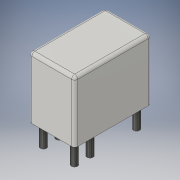
# Autodesk Inventor part: G5V-1-DC5_Relay
Saved by Autodesk Inventor 2016 (Build 200138000, 138)
## iProperties
Created: 2016-09-07
Part Number: G5V-1-DC5_Relay
Material: Generic
Document SubType Name: Modeling
Designer: jfixelle
Density: 1 g/cm^3
Appearance: White
Author: jfixelle
Autodesk Inventor part; units mm, degrees
ref_plane "YZ Plane" through (0, 0, 0) normal (1, 0, 0) x (0, 1, 0)
ref_plane "XZ Plane" through (0, 0, 0) normal (0, 1, 0) x (-1, 0, 0)
ref_plane "XY Plane" through (0, 0, 0) normal (0, 0, 1) x (1, 0, 0)
sketch "Sketch1" plane through (0, 0, 0) normal (0, 1, 0) x (-1, 0, 0)
  line L0 (3.75, 6.25) -> (-3.75, 6.25)
  line L1 (-3.75, 6.25) -> (-3.75, -6.25)
  line L2 (-3.75, -6.25) -> (3.75, -6.25)
  line L3 (3.75, -6.25) -> (3.75, 6.25)
  point P0 (0, 0)
  dimension "d0" = 7.5
  dimension "d1" = 3.75
  dimension "d2" = 12.5
  dimension "d3" = 6.25
  constraints: 8 end point, 2 parallel, 1 horizontal, 1 perpendicular
  measures "d0" distance of L1.end L2.end
  measures "d1" distance from line of point (0, 0) L3
  measures "d2" distance of L2.end L0.start
  measures "d3" distance from line of point (0, 0) L2
extrude "Extrusion1" add sketch "Sketch1" along normal blind 10
fillet "Fillet1" radius 0.5 8 edges at (3.75, 5, -6.25) (3.75, 5, 6.25) (-3.75, 5, 6.25) (0, 10, 6.25) (3.75, 10, 0) (0, 10, -6.25) (-3.75, 10, 0) (-3.75, 5, -6.25)
sketch "Sketch2" plane through (0, 0, 0) normal (0, -1, 0) x (1, 0, 0)
  circle A0 centre (2.54, 5.08) radius 0.5
  line L0 (3.75, 5.75) -> (3.75, -5.75) projected
  line L1 (3.75, 1.9877) -> (3.75, 0.9043)
  line L2 (1.2566, 6.25) -> (0.5094, 6.25)
  line L3 (-3.25, 6.25) -> (3.25, 6.25) projected
  circle A1 centre (2.54, 2.54) radius 0.5
  circle A2 centre (2.54, 0) radius 0.5
  circle A3 centre (2.54, -2.54) radius 0.5
  circle A4 centre (2.54, -5.08) radius 0.5
  circle A5 centre (-2.54, 5.08) radius 0.5
  circle A6 centre (-2.54, 2.54) radius 0.5
  circle A7 centre (-2.54, 0) radius 0.5
  circle A8 centre (-2.54, -2.54) radius 0.5
  circle A9 centre (-2.54, -5.08) radius 0.5
  point P0 (0, 0)
  dimension "d7" = 1
  dimension "d8" = 2.54
  dimension "d9" = 5.08
  dimension "d12" = 2.54
  dimension "d15" = 5.08
  constraints: 10 centre point, 4 end point, 3 point on line, 1 horizontal, 1 vertical, 18 other
  measures "d7" diameter of A0
  measures "d8" horizontal distance of point (0, 0) A0.centre
  measures "d9" vertical distance of point (0, 0) A0.centre
  measures "d12" distance of A0.centre A1.centre
  measures "d15" distance of A0.centre A5.centre
extrude "Extrusion2" add sketch "Sketch2" along normal blind 3.5 contours A0 | A1 | A4 | A5 | A6 | A9
body "Solid1"
